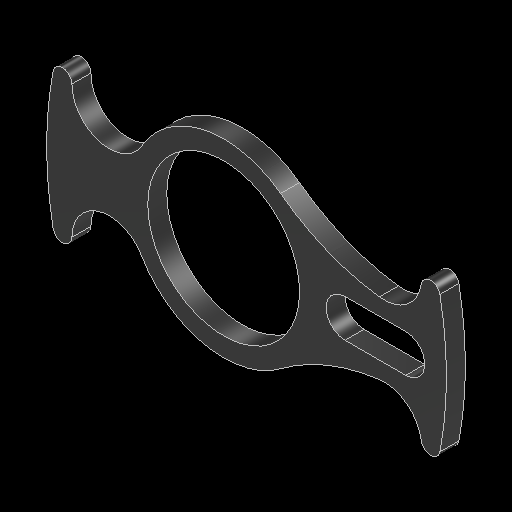
# Autodesk Inventor part: ShufflerFoot
Saved by Autodesk Inventor 2023 (Build 270158000, 158)
## iProperties
Created: 2022-03-05
Part Number: ShufflerFoot
Material: UHMW, Black
Document SubType Name: Modeling
Designer: tandu
Density: 0.94 g/cm^3
Appearance: Glossy - Black
Mass: 2.27555 g
Surface Area: 25.6077 cm^2
Volume: 2.42079 cm^3
Author: tandu
Autodesk Inventor part; units mm, degrees
ref_plane "YZ Plane" through (0, 0, 0) normal (1, 0, 0) x (0, 1, 0)
ref_plane "XZ Plane" through (0, 0, 0) normal (0, 1, 0) x (-1, 0, 0)
ref_plane "XY Plane" through (0, 0, 0) normal (0, 0, 1) x (1, 0, 0)
sketch "Sketch1" plane through (0, 0, 0) normal (0, 0, 1) x (1, 0, 0)
  circle A0 centre (0, 0) radius 12.7
  line L0 (30.48, 0) -> (20.32, 0) construction
  line L1 (30.48, 3.175) -> (20.32, 3.175)
  line L2 (20.32, -3.175) -> (30.48, -3.175)
  arc A1 (30.48, -3.175) -> (30.48, 3.175) centre (30.48, 0) ccw
  arc A2 (20.32, 3.175) -> (20.32, -3.175) centre (20.32, 0) ccw
  circle A3 centre (0, 0) radius 15.875
  line L3 (30.48, -5.715) -> (20.32, -5.715)
  arc A4 (20.32, 5.715) -> (20.32, -5.715) centre (20.32, 0) ccw
  line L4 (20.32, 5.715) -> (30.48, 5.715)
  arc A5 (30.48, -5.715) -> (30.48, 5.715) centre (30.48, 0) ccw
  line L5 (-15.875, 0) -> (-28.575, 0) construction
  line L6 (-28.575, -12.7) -> (-28.575, 12.7) construction
  line L7 (-26.9875, 11.1125) -> (-26.9875, -11.1125) construction
  line L8 (-28.575, 11.1125) -> (-28.575, -11.1125)
  line L9 (-25.4, -11.1125) -> (-25.4, 11.1125) construction
  arc A6 (-25.4, 11.1125) -> (-28.575, 11.1125) centre (-26.9875, 11.1125) ccw
  arc A7 (-28.575, -11.1125) -> (-25.4, -11.1125) centre (-26.9875, -11.1125) ccw
  arc A8 (-25.4, 11.1125) -> (-13.7291, 7.9703) centre (-19.1416, 11.1125) ccw
  arc A9 (-13.7291, -7.9703) -> (-25.4, -11.1125) centre (-19.1416, -11.1125) ccw
  arc A10 (30.48, -5.715) -> (9.525, -12.7) centre (30.48, -40.64) ccw
  arc A11 (9.525, 12.7) -> (30.48, 5.715) centre (30.48, 40.64) ccw
  arc A12 (-28.5461, 11.4139) -> (-28.5461, -11.4139) centre (30.48, 0) ccw
  line L10 (0, 0) -> (0, 12.7) construction
  arc A13 (36.195, -11.4139) -> (36.195, 11.4139) centre (-22.8311, 0) ccw
  line L11 (36.195, 11.4139) -> (36.195, -11.4139) construction
  circle A14 centre (34.6364, 11.1125) radius 1.5875 construction
  circle A15 centre (34.6364, -11.1125) radius 1.5875 construction
  arc A16 (33.0643, -11.333) -> (26.0776, -5.9936) centre (26.8665, -12.2021) ccw
  arc A17 (26.0776, 5.9936) -> (33.0643, 11.333) centre (26.8665, 12.2021) ccw
  arc A18 (36.195, 11.4139) -> (33.0643, 11.333) centre (34.6364, 11.1125) ccw
  arc A19 (33.0643, -11.333) -> (36.195, -11.4139) centre (34.6364, -11.1125) ccw
  point P0 (25.4, 0)
  point P1 (-26.9875, 0)
  point P2 (-26.9875, -12.7)
  point P3 (36.195, 0)
  dimension "d0" = 25.4
  dimension "d1" = 6.35
  dimension "d3" = 3.175
  dimension "d4" = 2.54
  dimension "d5" = 12.7
  dimension "d6" = 25.4
  dimension "d7" = 3.175
  dimension "d11" = 10.16
  dimension "d12" = 25.4
  constraints: 47 point on circle, 28 end point, 26 tangent, 19 centre point, 7 equal radius, 4 horizontal alignment, 4 midpoint, 4 vertical, 3 parallel, 2 coincident, 2 horizontal, 2 point on line, 2 vertical alignment, 5 other
  measures "d1" diameter of A2
  measures "d4" distance between parallel lines of L2 L3
  measures "d5" distance of L5.end L5.start
  measures "d6" distance of L6.start L6.end
  measures "d7" diameter of A7
  measures "d11" distance of L0.end L0.start
  measures "d12" distance of point (25.4, 0) point (0, 0)
extrude "Extrusion1" add sketch "Sketch1" along normal blind 3.175
equation "\"d0\" = CamSize1"
equation "\"d1\" = TopStandoffDiameter"
equation "\"d11\" = 2 * Offset1"
equation "\"d12\" = TopStandoffOffset1"
equation "\"CamSize1\" = 25.4"
equation "\"TopStandoffDiameter\" = 6.35"
equation "\"Offset1\" = 5.08"
equation "\"TopStandoffOffset1\" = 25.4"
body "Solid1"
